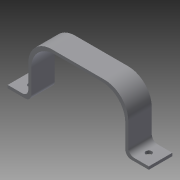
# Autodesk Inventor part: hendel
Saved by Autodesk Inventor 2015 (Build 190159000, 159)
## iProperties
Created: 2015-01-22
Part Number: hendel
Material: Generic
Document SubType Name: Modeling
Designer: 215152
Density: 1 g/cm^3
Appearance: Default
Author: 215152
Autodesk Inventor part; units mm, degrees
ref_plane "YZ Plane" through (0, 0, 0) normal (1, 0, 0) x (0, 1, 0)
ref_plane "XZ Plane" through (0, 0, 0) normal (0, 1, 0) x (-1, 0, 0)
ref_plane "XY Plane" through (0, 0, 0) normal (0, 0, 1) x (1, 0, 0)
sketch "Sketch1" plane through (0, 0, 0) normal (0, 0, 1) x (1, 0, 0)
  line L0 (0, 0) -> (101.6, 0) construction
  line L1 (101.6, 0) -> (101.6, 38.1) construction
  line L2 (101.6, 38.1) -> (0, 38.1) construction
  line L3 (0, 38.1) -> (0, 0) construction
  line L4 (0, 0) -> (19.05, 0)
  line L5 (101.6, 0) -> (82.55, 0)
  line L6 (25.4, 6.35) -> (25.4, 15.875)
  line L7 (38.1, 28.575) -> (63.5, 28.575)
  line L8 (76.2, 15.875) -> (76.2, 6.35)
  line L9 (66.675, 31.75) -> (34.925, 31.75)
  line L10 (22.225, 19.05) -> (22.225, 9.525)
  line L11 (15.875, 3.175) -> (0, 3.175)
  line L12 (101.6, 3.175) -> (85.725, 3.175)
  line L13 (79.375, 9.525) -> (79.375, 19.05)
  line L14 (0, 0) -> (0, 3.175)
  line L15 (101.6, 0) -> (101.6, 3.175)
  arc A0 (34.925, 31.75) -> (22.225, 19.05) centre (34.925, 19.05) ccw
  arc A1 (38.1, 28.575) -> (25.4, 15.875) centre (38.1, 15.875) ccw
  arc A2 (79.375, 19.05) -> (66.675, 31.75) centre (66.675, 19.05) ccw
  arc A3 (76.2, 15.875) -> (63.5, 28.575) centre (63.5, 15.875) ccw
  arc A4 (15.875, 3.175) -> (22.225, 9.525) centre (15.875, 9.525) ccw
  arc A5 (79.375, 9.525) -> (85.725, 3.175) centre (85.725, 9.525) ccw
  arc A6 (76.2, 6.35) -> (82.55, 0) centre (82.55, 6.35) ccw
  arc A7 (19.05, 0) -> (25.4, 6.35) centre (19.05, 6.35) ccw
  point P0 (25.4, 0)
  point P1 (76.2, 0)
  point P2 (25.4, 28.575)
  dimension "d0" = 101.6
  dimension "d1" = 38.1
  dimension "d2" = 25.4
  dimension "d3" = 25.4
  dimension "d4" = 28.575
  dimension "d5" = 3.175
  dimension "d6" = 3.175
  dimension "d7" = 12.7
  dimension "d8" = 6.35
  dimension "d9" = 6.35
  dimension "d10" = 6.35
  constraints: 32 end point, 16 point on circle, 16 tangent, 10 point on line, 8 centre point, 6 perpendicular, 4 equal radius, 2 collinear, 2 parallel, 1 horizontal, 1 vertical, 3 other
  measures "d0" distance of L2.end L1.end
  measures "d1" distance of L1.end L0.end
  measures "d2" distance of L0.start point (25.4, 0)
  measures "d3" distance of L0.end point (76.2, 0)
  measures "d4" distance of point (25.4, 0) point (25.4, 28.575)
  measures "d5" distance between parallel lines of L6 L10
  measures "d6" distance between parallel lines of L8 L13
  measures "d7" radius of A0
  measures "d8" radius of A4
  measures "d9" radius of A5
  measures "d10" radius of A7
extrude "Extrusion1" add sketch "Sketch1" along normal blind 25.4
sketch "Sketch2" plane through (0, 0, 0) normal (0, -1, 0) x (1, 0, 0)
  line L0 (0, 0) -> (19.05, 0) projected
  line L1 (19.05, 0) -> (19.05, 25.4) projected
  line L2 (0, 25.4) -> (19.05, 25.4) projected
  line L3 (0, 0) -> (0, 25.4) projected
  line L4 (82.55, 0) -> (101.6, 0) projected
  line L5 (101.6, 0) -> (101.6, 25.4) projected
  line L6 (82.55, 25.4) -> (101.6, 25.4) projected
  line L7 (82.55, 0) -> (82.55, 25.4) projected
  point P0 (12.7, 12.7)
  point P1 (88.9, 12.7)
  dimension "d13" = 12.7
  dimension "d14" = 12.7
  dimension "d15" = 12.7
  dimension "d16" = 12.7
  measures "d13" distance from line of L3 point (12.7, 12.7)
  measures "d14" distance from line of L0 point (12.7, 12.7)
  measures "d15" distance from line of L4 point (88.9, 12.7)
  measures "d16" distance from line of L5 point (88.9, 12.7)
hole "Hole1" at (12.7, 0, 12.7) at (88.9, 0, 12.7) direction (0, 1, 0) diameter 6.35 end through all
fillet "Fillet1" radius 3.175 4 edges at (101.6, 1.5875, 25.4) (101.6, 1.5875, 0) (0, 1.5875, 25.4) (0, 1.5875, 0)
body "Solid1"
